Diaper Place (Autodesk Fusion 360 design; units mm, degrees)
Autodesk Fusion 360 part; units mm, degrees
sketch "Sketch1" plane through (0, 0, 0) normal (0, 0, 1) x (1, 0, 0)
  line L0 (0, 0) -> (1615, 0)
  line L1 (1615, 0) -> (1615, 505)
  line L2 (1615, 505) -> (0, 505)
  line L3 (0, 505) -> (0, 0)
  line L4 (50, 493) -> (1565, 493)
  line L5 (1565, 493) -> (1565, 15)
  line L6 (1565, 15) -> (50, 15)
  line L7 (50, 15) -> (50, 493)
  dimension "d1" = 505
  dimension "d2" = 1615
  dimension "d3" = 12
  dimension "d4" = 50
  dimension "d5" = 50
  dimension "d6" = 15
  constraint horizontal L0
  constraint vertical L1
  constraint horizontal L2
  constraint vertical L3
  constraint coincident L0.start L3.end
  constraint horizontal L4
  constraint vertical L5
  constraint horizontal L6
  constraint vertical L7
  measures "d1" distance of L0.start L2.end
  measures "d2" distance of L1.end L2.end
  measures "d3" distance of L2 L4
  measures "d4" distance of L3 L7
  measures "d5" distance of L1 L5
  measures "d6" distance of L0 L6
extrude "Extrude1" add sketch "Sketch1" along normal blind 23 contours L0 L1 L2 L3 | L4 L5 L6 L7 makes body 1
extrude "Extrude2" add sketch "Sketch1" against normal blind 942 contours L4 L5 L6 L7 bodies 1
sketch "Sketch2" plane through (0, 0, 23) normal (0, 0, 1) x (-1, 0, 0)
  line L0 (0, -505) -> (0, 0)
  line L1 (0, 0) -> (-1615, 0)
  line L2 (-1615, 0) -> (-1615, -505)
  line L3 (-1615, -505) -> (0, -505)
  line L4 (-517.9302, -505) -> (-1367.9302, -505)
  line L5 (-1367.9302, -505) -> (-1367.9302, 255)
  line L6 (-1367.9302, 255) -> (-517.9302, 255)
  line L7 (-517.9302, 255) -> (-517.9302, -505)
  line L8 (-1615, -505) -> (0, -505)
  line L9 (-517.9302, -115) -> (-1367.9302, -115)
  dimension "d11" = 850
  dimension "d12" = 760
  dimension "d15" = 390
  constraint horizontal L4
  constraint vertical L5
  constraint horizontal L6
  constraint vertical L7
  constraint coincident L4.start L8
  constraint coincident L7 L9.start
  constraint coincident L5 L9.end
  constraint perpendicular L5 L9
  measures "d11" distance of L4.start L4.end
  measures "d12" distance of L4.start L6.end
  measures "d15" distance of L4 L9
extrude "Extrude3" add sketch "Sketch2" along normal blind 15 separate body contours L3 L4 L5 L7 L8 L9 makes body 2
extrude "Extrude4" add sketch "Sketch2" along normal blind 15 separate body contours L1 L5 L7 L9 | L1 L5 L6 L7 makes body 3
sketch "Sketch3" plane through (1367.9302, 0, 0) normal (1, 0, 0) x (0, 1, 0)
  line L0 (115, 23) -> (505, 23)
  line L1 (505, 23) -> (505, 38)
  line L2 (505, 38) -> (115, 38)
  line L3 (115, 38) -> (115, 23)
  line L4 (505, 23) -> (-255, 23)
  line L5 (-255, 23) -> (-255, 108)
  line L6 (-255, 108) -> (505, 108)
  line L7 (505, 108) -> (505, 23)
  dimension "d21" = 760
  dimension "d22" = 85
  constraint horizontal L4
  constraint vertical L5
  constraint horizontal L6
  constraint vertical L7
  constraint coincident L0.end L1.start
  measures "d21" distance of L0.end L4.end
  measures "d22" distance of L0.end L6.end
extrude "Extrude5" add sketch "Sketch3" along normal blind 15 separate body makes body 4
extrude "Extrude6" add sketch "Sketch3" along normal blind 15 from surface at -865 separate body makes body 5
sketch "Sketch6" plane through (0, 505, 0) normal (0, 1, 0) x (-1, 0, 0)
  line L0 (-1615, 0) -> (0, 0)
  line L1 (0, 0) -> (0, 23)
  line L2 (0, 23) -> (-1615, 23)
  line L3 (-1615, 23) -> (-1615, 0)
  line L4 (-1382.9302, 108) -> (-502.9302, 108)
  line L5 (-502.9302, 108) -> (-502.9302, -15)
  line L6 (-502.9302, -15) -> (-1382.9302, -15)
  line L7 (-1382.9302, -15) -> (-1382.9302, 108)
  point P0 (-1382.9302, 108)
  point P1 (-502.9302, 108)
  dimension "d29" = 15
  constraint horizontal L4
  constraint vertical L5
  constraint horizontal L6
  constraint vertical L7
  constraint coincident P0 L4.start
  constraint coincident P1 L4.end
  measures "d29" distance of L0 L6
extrude "Extrude7" add sketch "Sketch6" along normal blind 15 separate body contours L0 L2 L5 L7 | L0 L5 L6 L7 | L2 L4 L5 L7 makes body 6
fillet "Fillet1" radius 85 2 edges at (1375.4302, -255, 108) (510.4302, -255, 108) on bodies 4 5
copy_body "Body->Comp1" bodies 2 removing the originals makes body 7 in component "base back"
copy_body "Body->Comp2" bodies 3 removing the originals makes body 8 in component "base front"
component "base back" placed x (1, 0, 0) y (0, 1, 0) z (0, 0, 1) at (0, 0, 0)
component "base front" placed x (1, 0, 0) y (0, 1, 0) z (0, 0, 1) at (0, 0, 0)
equation "d11 = base_width"
equation "d12 = base_height"
equation "base_width = 850 mm"
equation "base_height = 760 mm"
equation "d15 = base_height / 2 + 10 mm"
equation "material_thickness = 15 mm"
equation "d17 = material_thickness"
equation "d19 = material_thickness"
equation "d21 = base_height"
equation "d22 = base_sidewalls - material_thickness"
equation "base_sidewalls = 100 mm"
equation "d24 = material_thickness"
equation "d26 = -( base_width + material_thickness )"
equation "d27 = material_thickness"
equation "d29 = material_thickness"
equation "d30 = material_thickness"
equation "d33 = base_sidewalls - material_thickness"
named bodies: "Schrank", "base back", "base front", "base side right", "base side left", "base side back"
